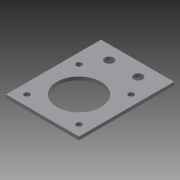
# Autodesk Inventor part: NEMA 23 Holder
Saved by Autodesk Inventor 2015 (Build 190159000, 159)
## iProperties
Created: 2017-01-20
Part Number: NEMA 23 Holder
Material: Generic
Document SubType Name: Modeling
Designer: Guy
Density: 1 g/cm^3
Appearance: Default
Author: Guy
Autodesk Inventor part; units mm, degrees
ref_plane "YZ Plane" through (0, 0, 0) normal (1, 0, 0) x (0, 1, 0)
ref_plane "XZ Plane" through (0, 0, 0) normal (0, 1, 0) x (-1, 0, 0)
ref_plane "XY Plane" through (0, 0, 0) normal (0, 0, 1) x (1, 0, 0)
sketch "Sketch1" plane through (0, 0, 0) normal (0, 0, 1) x (1, 0, 0)
  circle A0 centre (0, 0) radius 20
  line L0 (-33.2, 28.2) -> (33.2, 28.2)
  line L1 (33.2, 28.2) -> (33.2, -33.2)
  line L2 (33.2, -33.2) -> (-33.2, -33.2)
  line L3 (-33.2, -33.2) -> (-33.2, 28.2)
  circle A1 centre (-23.7, 23.7) radius 2.5
  circle A2 centre (23.7, 23.7) radius 2.5
  circle A3 centre (23.7, -23.7) radius 2.5
  circle A4 centre (-23.7, -23.7) radius 2.5
  line L4 (-33.2, 28.2) -> (-33.2, 53.2)
  line L5 (-33.2, 53.2) -> (33.2, 53.2)
  line L6 (33.2, 53.2) -> (33.2, 28.2)
  circle A5 centre (-13.2, 40.7) radius 4
  circle A6 centre (13.2, 40.7) radius 4
  dimension "d0" = 40
  dimension "d1" = 66.4
  dimension "d2" = 61.4
  dimension "d3" = 33.2
  dimension "d4" = 28.2
  dimension "d5" = 5
  dimension "d6" = 5
  dimension "d7" = 5
  dimension "d8" = 5
  dimension "d9" = 47.4
  dimension "d10" = 47.4
  dimension "d11" = 47.4
  dimension "d12" = 47.4
  dimension "d13" = 4.5
  dimension "d14" = 9.5
  dimension "d15" = 9.5
  dimension "d16" = 9.5
  dimension "d19" = 25
  dimension "d20" = 8
  dimension "d21" = 8
  dimension "d23" = 20
  dimension "d24" = 20
  dimension "d25" = 12.5
  dimension "d26" = 12.5
  constraints: 14 end point, 7 centre point, 3 perpendicular, 2 parallel, 1 coincident, 1 horizontal, 1 vertical
  measures "d0" diameter of A0
  measures "d1" distance between parallel lines of L1 L3
  measures "d2" distance between parallel lines of L2 L0
  measures "d3" distance from line of point (0, 0) L1
  measures "d4" distance from line of point (0, 0) L0
  measures "d5" diameter of A2
  measures "d6" diameter of A3
  measures "d7" diameter of A4
  measures "d8" diameter of A1
  measures "d9" distance of A1.centre A2.centre
  measures "d10" distance of A3.centre A4.centre
  measures "d11" distance of A1.centre A4.centre
  measures "d12" distance of A3.centre A2.centre
  measures "d13" distance from line of A1.centre L0
  measures "d14" distance from line of L3 A1.centre
  measures "d15" distance from line of L1 A3.centre
  measures "d16" distance from line of L2 A3.centre
  measures "d19" distance between parallel lines of L0 L5
  measures "d20" diameter of A6
  measures "d21" diameter of A5
  measures "d23" distance from line of L6 A6.centre
  measures "d24" distance from line of L4 A5.centre
  measures "d25" distance from line of L0 A6.centre
  measures "d26" distance from line of L0 A5.centre
extrude "Extrusion1" add sketch "Sketch1" along normal blind 3
body "Solid1"
